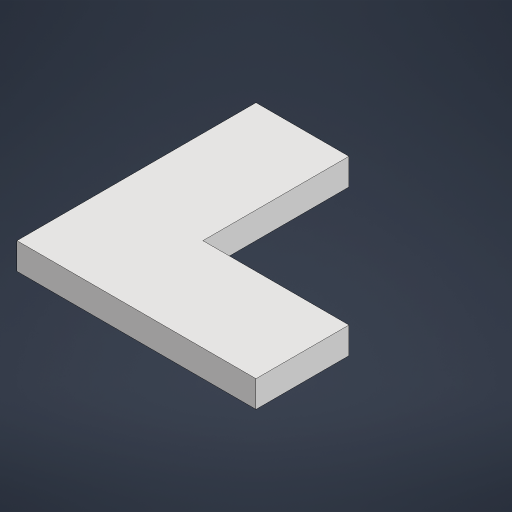
# Autodesk Inventor part: L - 6
Saved by Autodesk Inventor 2023.2 (Build 272271000, 271)
## iProperties
Created: 2022-11-30
Part Number: L - 6
Material: Generic
Document SubType Name: Modeling
Designer: awelt
Mass: 6653.15 g
Surface Area: 3548.38 cm^2
Volume: 6653.15 cm^3
Density: 1 g/cm^3
Appearance: Default
RuleStatus: InUse
BeforeDocSave0: file://C:\Users\awelt\Documents\Inventor\iLogic_Rules\BoundingStore
DocClose0: file://C:\Users\awelt\Documents\Inventor\iLogic_Rules\BoundingStore
Author: awelt
BoundingBL1: 2
BoundingBL2: 18
BoundingBL3: 18
BoundingCF: 0.375
Autodesk Inventor part; units mm, degrees
ref_plane "YZ Plane" through (0, 0, 0) normal (1, 0, 0) x (0, 1, 0)
ref_plane "XZ Plane" through (0, 0, 0) normal (0, 1, 0) x (-1, 0, 0)
ref_plane "XY Plane" through (0, 0, 0) normal (0, 0, 1) x (1, 0, 0)
sketch "Sketch2" plane through (0, 0, 0) normal (0, 1, 0) x (-1, 0, 0)
  line L0 (0, -457.2) -> (0, 0)
  line L1 (0, 0) -> (-457.2, 0)
  line L2 (-177.8, -457.2) -> (-177.8, -177.8)
  line L3 (-177.8, -177.8) -> (-457.2, -177.8)
  line L4 (-177.8, -457.2) -> (0, -457.2)
  line L5 (-457.2, -177.8) -> (-457.2, 0)
  dimension "d3" = 457.2
  dimension "d4" = 177.8
  constraints: 12 end point, 4 perpendicular, 1 horizontal, 1 vertical, 1 other
  measures "d3" distance of L0.start L0.end
  measures "d4" distance between parallel lines of L0 L2
extrude "Extrusion1" add sketch "Sketch2" along normal blind 50.8
body "Solid1"
